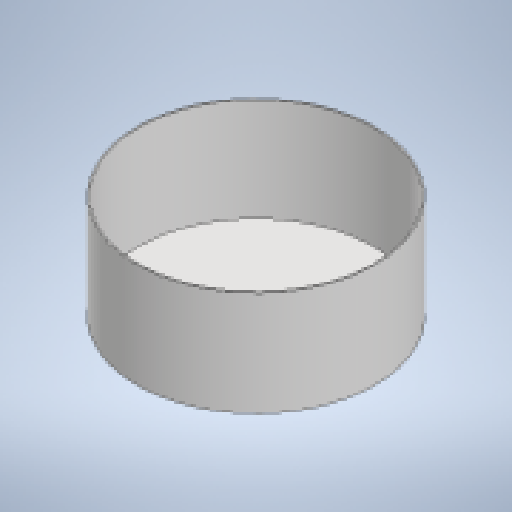
# Autodesk Inventor part: Cuenco
Saved by Autodesk Inventor 2024 (Build 280153000, 153)
## iProperties
Created: 2024-07-17
Part Number: Cuenco
Material: Genérico
Document SubType Name: Modeling
Designer: sergi
Density: 1 g/cm^3
Appearance: Valor por defecto
Author: sergi
Autodesk Inventor part; units mm, degrees
ref_plane "YZ Plane" through (0, 0, 0) normal (1, 0, 0) x (0, 1, 0)
ref_plane "XZ Plane" through (0, 0, 0) normal (0, 1, 0) x (-1, 0, 0)
ref_plane "XY Plane" through (0, 0, 0) normal (0, 0, 1) x (1, 0, 0)
sketch "Boceto1" plane through (0, 0, 0) normal (0, 1, 0) x (-1, 0, 0)
  circle A0 centre (0, 0) radius 80
  circle A1 centre (0, 0) radius 52.5
  dimension "d0" = 160
  dimension "d4" = 105
  constraints: 2 centre point, 2 coincident
  measures "d0" diameter of A0
  measures "d4" diameter of A1
extrude "Extrusión1" add sketch "Boceto1" along normal blind 25 draft 50 contours A1
shell "Vaciado1" thickness 3 removed faces 1 at (12.2178, 25, 3.7687)
